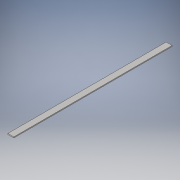
# Autodesk Inventor part: mirror
Saved by Autodesk Inventor 2016 (Build 200138000, 138)
## iProperties
Created: 2015-12-05
Part Number: mirror
Material: Glass
Document SubType Name: Modeling
Designer: acd
Density: 2.18 g/cm^3
Appearance: Clear
Author: acd
Autodesk Inventor part; units mm, degrees
ref_plane "YZ Plane" through (0, 0, 0) normal (1, 0, 0) x (0, 1, 0)
ref_plane "XZ Plane" through (0, 0, 0) normal (0, 1, 0) x (-1, 0, 0)
ref_plane "XY Plane" through (0, 0, 0) normal (0, 0, 1) x (1, 0, 0)
sketch "Sketch1" plane through (0, 0, 0) normal (0, 1, 0) x (-1, 0, 0)
  line L0 (-15, 400) -> (15, 400)
  line L1 (15, 400) -> (15, -400)
  line L2 (15, -400) -> (-15, -400)
  line L3 (-15, -400) -> (-15, 400)
  line L4 (-15, 400) -> (15, -400) construction
  line L5 (15, 400) -> (-15, -400) construction
  point P0 (0, 0)
  dimension "d0" = 30
  dimension "d1" = 800
  constraints: 12 end point, 2 midpoint, 2 parallel, 1 horizontal, 1 perpendicular
  measures "d0" distance of L1.end L2.end
  measures "d1" distance of L0.end L1.end
extrude "Extrusion1" add sketch "Sketch1" along normal blind 5
body "Solid1"
